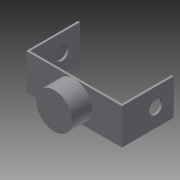
# Autodesk Inventor part: Sholder_Pitch
Saved by Autodesk Inventor 2013 (Build 170138000, 138)
## iProperties
Created: 2012-12-03
Part Number: Sholder_Pitch
Material: Generic
Document SubType Name: Modeling
Designer: Joe
Density: 1 g/cm^3
Author: Joe
Autodesk Inventor part; units mm, degrees
ref_plane "YZ Plane" through (0, 0, 0) normal (1, 0, 0) x (0, 1, 0)
ref_plane "XZ Plane" through (0, 0, 0) normal (0, 1, 0) x (-1, 0, 0)
ref_plane "XY Plane" through (0, 0, 0) normal (0, 0, 1) x (1, 0, 0)
sketch "Sketch1" plane through (0, 0, 0) normal (0, 0, 1) x (1, 0, 0)
  line L0 (0, 0) -> (27, 0) construction
  line L1 (27, 0) -> (27, 27)
  line L2 (27, 27) -> (0, 27)
  line L3 (0, 27) -> (0, 0) construction
  line L4 (-27, 0) -> (-27, 27)
  line L5 (-27, 27) -> (0, 27)
  line L6 (27, 0) -> (27, -27)
  line L7 (27, -27) -> (0, -27)
  line L8 (-27, -27) -> (0, -27)
  line L9 (-27, 0) -> (-27, -27)
  dimension "d0" = 27
  constraints: 20 end point, 5 symmetric about line, 2 parallel, 2 perpendicular, 1 horizontal
  measures "d0" distance of L1.end L2.end
extrude "Extrusion1" add sketch "Sketch1" along normal mid plane 138
sketch "Sketch2" plane through (0, 0, 69) normal (0, 0, 1) x (1, 0, 0)
  line L0 (27, -27) -> (27, 27) projected
  line L1 (27, 27) -> (-27, 27) projected
  line L2 (-27, 27) -> (-27, -27) projected
  line L3 (-27, -27) -> (27, -27) projected
  circle A0 centre (0, 0) radius 27
  constraints: 1 centre point, 1 coincident
extrude "Extrusion2" cut sketch "Sketch2" against normal blind 30 contours L3 A0 L0 | A0 L1 L0 | L3 L2 A0 | A0 L2 L1
sketch "Sketch3" plane through (0, 0, 69) normal (0, 0, 1) x (1, 0, 0)
  circle A0 centre (0, 0) radius 27 projected
  line L0 (-51, 27) -> (27, 27)
  line L1 (27, 27) -> (27, -27)
  line L2 (27, -27) -> (-51, -27)
  line L3 (-51, -27) -> (-51, 27)
  line L4 (27, 27) -> (27, 0) projected
  line L5 (27, 27) -> (27, -27) projected
  line L6 (0, 27) -> (27, 27) projected
  line L7 (27, -27) -> (0, -27) projected
  dimension "d6" = 51
  constraints: 8 end point, 3 collinear, 2 parallel, 1 horizontal, 1 perpendicular
  measures "d6" distance from line of A0.centre L3
extrude "Extrusion3" add sketch "Sketch3" along normal blind 3
sketch "Sketch4" plane through (0, 0, 72) normal (0, 0, 1) x (1, 0, 0)
  circle A0 centre (0, 0) radius 10
  dimension "d9" = 20
  constraints: 1 centre point, 1 coincident
  measures "d9" diameter of A0
extrude "Extrusion4" cut sketch "Sketch4" against normal blind 3
mirror "Mirror1" about plane through (0, 0, 0) normal (0, 0, 1) of "Extrusion3", "Extrusion4"
sketch "Sketch5" plane through (-51, 27, -69) normal (0, 0, 1) x (1, 0, 0)
  line L0 (24, -54) -> (0, -54) projected
  line L1 (0, 0) -> (3, 0)
  line L2 (3, 0) -> (3, -54)
  line L3 (3, -54) -> (0, -54)
  line L4 (0, -54) -> (0, 0)
  point P0 (51, -27)
  dimension "d13" = 3
  constraints: 8 end point, 2 parallel, 1 horizontal, 1 perpendicular, 1 point on line
  measures "d13" distance between parallel lines of L2 L4
extrude "Extrusion5" add sketch "Sketch5" along normal up to next
sketch "Sketch6" plane through (-51, -27, 72) normal (-1, 0, 0) x (0, 0, 1)
  line L0 (0, 0) -> (-144, 0) projected
  circle A0 centre (-72, 27) radius 27
  constraints: 1 centre point, 1 coincident, 1 tangent
extrude "Extrusion6" add sketch "Sketch6" along normal blind 30
sketch "Sketch7" plane through (-27, 27, 39) normal (0, 1, 0) x (1, 0, 0)
  line L0 (0, 108) -> (54, 108)
  line L1 (54, 108) -> (54, -30)
  line L2 (54, -30) -> (0, -30)
  line L3 (0, -30) -> (0, 108)
  point P0 (27, 39)
  constraints: 8 end point, 2 parallel, 1 horizontal, 1 perpendicular
extrude "Extrusion7" cut sketch "Sketch7" against normal through all
move or copy body "Move Body1" bodies to move or copy 1 copy no rotation origin (0, 0, 0) rotation axis (1, 0, 0) rotation angle 90
move or copy body "Move Body2" bodies to move or copy 1 copy no rotation origin (0, 0, 0) rotation axis (0, 0, 1) rotation angle 90
body "Solid1"
